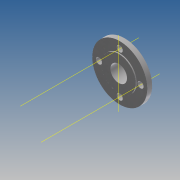
# Autodesk Inventor part: part
Saved by Autodesk Inventor 2016 (Build 200138000, 138)
## iProperties
Created: 2017-09-17
Part Number: part
Material: Steel, Cast
Document SubType Name: Modeling
Designer: Fauszt
Density: 7.85 g/cm^3
Appearance: Semi-Polished
Mass: 2721.5 g
Surface Area: 589.926 cm^2
Volume: 346.688 cm^3
Author: Fauszt
Autodesk Inventor part; units mm, degrees
ref_plane "YZ Plane" through (0, 0, 0) normal (1, 0, 0) x (0, 1, 0)
ref_plane "XZ Plane" through (0, 0, 0) normal (0, 1, 0) x (-1, 0, 0)
ref_plane "XY Plane" through (0, 0, 0) normal (0, 0, 1) x (1, 0, 0)
sketch "Sketch1" plane through (0, 0, 0) normal (1, 0, 0) x (0, 1, 0)
  line L0 (-9, 0) -> (54, 0) projected
  line L1 (0, -16.5) -> (0, 99) construction
  line L2 (45, 25) -> (0, 25)
  line L3 (0, 25) -> (0, 82.5)
  line L4 (0, 82.5) -> (18, 82.5)
  line L5 (18, 82.5) -> (18, 27.9)
  line L6 (18, 27.9) -> (45, 27.9)
  line L7 (45, 27.9) -> (45, 25)
  point P0 (0, 0)
  dimension "d0" = 165
  dimension "d45" = 45
  dimension "d46" = 50
  dimension "d47" = 18
  dimension "d48" = 2.9
  constraints: 12 end point, 4 perpendicular, 2 point on line, 1 vertical
  measures "d0" diameter of L4 L0
  measures "d45" distance between parallel lines of L3 L7
  measures "d46" diameter of L2 L0
  measures "d47" distance of L3.end L4.end
  measures "d48" distance of L6.end L2.start
revolve "Revolution1" add sketch "Sketch1" angle 360 about axis through (0, 0, 0) along (0, 1, 0)
sketch "Sketch2" plane through (0, 0, 0) normal (1, 0, 0) x (0, 1, 0)
  line L0 (0, -115.5) -> (0, 115.5) construction
  line L1 (0, 82.5) -> (18, 82.5) construction
  line L2 (3, 82.5) -> (3, 51)
  line L3 (3, 51) -> (0, 51)
  line L4 (-3.6, 0) -> (21.6, 0) projected
  line L5 (3, 82.5) -> (0, 82.5)
  line L6 (0, -82.5) -> (0, 82.5) projected
  line L7 (0, 82.5) -> (0, 51)
  point P0 (0, 0)
  dimension "d49" = 3
  dimension "d50" = 102
  constraints: 8 end point, 2 horizontal, 2 point on line, 1 collinear, 1 vertical
  measures "d49" distance between parallel lines of L0 L2
  measures "d50" diameter of L3 L4
revolve "Revolution2" cut sketch "Sketch2" angle 360 about axis through (0, -10, 0) along (0, 1, 0)
sketch "Sketch5" plane through (0, 18, 0) normal (0, 1, 0) x (1, 0, 0)
  line L0 (0, 115.5) -> (0, -115.5) construction
  point P0 (0, 0)
  point P1 (0, -62.5)
  dimension "d24" = 62.5
  constraints: 1 point on line
  measures "d24" distance of point (0, -62.5) point (0, 0)
hole "Hole3" at (0, 18, 62.5) direction (0, -1, 0) diameter 18 end through all
pattern_circular "Circular Pattern1" count 4 over 360 about axis through (0, -10, 0) along (0, 1, 0) of "Hole3"
sketch "Sketch6" plane through (0, 0, 0) normal (0, 0, 1) x (1, 0, 0)
  line L0 (82.5, 18) -> (-82.5, 18) construction
  line L1 (-27.9, 18) -> (-27.9, 45) construction
  line L2 (-27.9, 18) -> (-27.9, 37)
  line L3 (27.9, 18) -> (-27.9, 18) projected
  line L4 (-27.9, 18) -> (-46.9, 18)
  line L5 (0, -9) -> (0, 54) projected
  line L6 (-27.9, 37) -> (-46.9, 18)
  point P0 (0, 0)
  dimension "d52" = 8
  constraints: 6 end point, 2 point on line, 1 collinear, 1 perpendicular
  measures "d52" distance of L2.end L1.end
revolve "Revolution3" add sketch "Sketch6" angle 360 about axis through (0, -10, 0) along (0, 1, 0)
fillet "Fillet2" radius 6 1 edges at (46.9, 18, 0)
fillet "Fillet3" radius 0.2 15 edges at (0, 45, -25) (0, 18, -82.5) (0, 3, -82.5) (0, 0, -51) (0, 18, 53.5) (0, 3, 53.5) (0, 45, -27.9) (-19.7283, 37, 19.7283) (19.7283, 37, -19.7283) (53.5, 18, 0) (-53.5, 18, 0) (0, 18, -53.5) (-53.5, 3, 0) (53.5, 3, 0) (0, 3, -53.5)
equation "\"d0\" = D"
equation "\"d45\" = h1"
equation "\"d46\" = DN"
equation "\"d47\" = b"
equation "\"d48\" = ss"
equation "\"d49\" = fff"
equation "\"d50\" = d4"
equation "\"d24\" = 0.5 * k"
equation "\"d52\" = h2"
equation "\"DN\" = 50"
equation "\"D\" = 165"
equation "\"d1\" = 57"
equation "\"b\" = 18"
equation "\"k\" = 125"
equation "\"h1\" = 45"
equation "\"d3\" = 72"
equation "\"ss\" = 2.9"
equation "\"r\" = 6"
equation "\"h2\" = 8"
equation "\"d4\" = 102"
equation "\"fff\" = 3"
body "Solid1"
